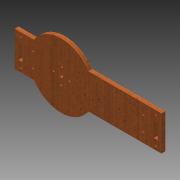
# Autodesk Inventor part: tiltStructureCrossBeamRB01
Saved by Autodesk Inventor 2013 (Build 170138000, 138)
## iProperties
Created: 2014-06-14
Part Number: tiltStructureCrossBeamRB01
Material: Wood (Cherry)
Document SubType Name: Modeling
Designer: Byron
Density: 0.5 g/cm^3
Mass: 49.6326 g
Surface Area: 357.646 cm^2
Volume: 99.2651 cm^3
Author: Byron
Autodesk Inventor part; units mm, degrees
ref_plane "YZ Plane" through (0, 0, 0) normal (1, 0, 0) x (0, 1, 0)
ref_plane "XZ Plane" through (0, 0, 0) normal (0, 1, 0) x (-1, 0, 0)
ref_plane "XY Plane" through (0, 0, 0) normal (0, 0, 1) x (1, 0, 0)
sketch "Sketch1" plane through (0, 0, 0) normal (0, 0, 1) x (1, 0, 0)
  line L0 (0, 78.0122) -> (0, 82.508) projected
  line L1 (-6.35, 82.508) -> (-6.35, 78.0122) projected
  line L2 (-6.35, 78.0122) -> (0, 78.0122) projected
  line L3 (222.25, 130.6664) -> (222.25, 135.1622) projected
  line L4 (215.9, 135.1622) -> (222.25, 135.1622) projected
  line L5 (215.9, 135.1622) -> (215.9, 130.6664) projected
  line L6 (222.25, 78.0122) -> (222.25, 135.1622)
  line L7 (-6.35, 135.1622) -> (-6.35, 78.0122)
  arc A0 (65.1726, 108.6235) -> (63.7223, 104.0872) centre (63.7223, 106.5872) ccw projected
  line L8 (222.25, 135.1622) -> (108.3945, 135.1622)
  line L9 (19.05, 135.1622) -> (-6.35, 135.1622)
  line L10 (-6.35, 78.0122) -> (19.05, 78.0122)
  line L11 (108.3945, 78.0122) -> (222.25, 78.0122)
  arc A1 (108.3945, 135.1622) -> (19.05, 135.1622) centre (63.7223, 106.5872) ccw
  arc A2 (19.05, 78.0122) -> (108.3945, 78.0122) centre (63.7223, 106.5872) ccw
  line L12 (215.9, 130.6664) -> (222.25, 130.6664) projected
  line L13 (0, 82.508) -> (-6.35, 82.508) projected
  point P0 (0, 0)
  dimension "d19" = 57.15
  dimension "d20" = 57.15
  dimension "d21" = 228.6
  dimension "d22" = 228.6
  dimension "d23" = 25.4
  dimension "d24" = 25.4
  dimension "d25" = 113.8555
  dimension "d26" = 113.8555
  constraints: 12 end point, 5 parallel, 4 point on circle, 2 centre point, 2 horizontal, 2 perpendicular, 1 coincident
  measures "d19" distance of L6.start L3.end
  measures "d20" distance of L7.start L1.end
  measures "d21" distance of L6.start L1.end
  measures "d22" distance of L3.end L7.start
  measures "d23" distance of L9.start L7.start
  measures "d24" distance of L1.end L10.end
  measures "d25" distance of L3.end L8.end
  measures "d26" distance of L11.start L6.start
extrude "Extrusion1" add sketch "Sketch1" along normal blind 6.35
sketch "Sketch2" plane through (0, 0, 0) normal (0, 0, -1) x (-1, 0, 0)
  line L0 (-53.2456, 114.8496) -> (-74.1989, 114.8496)
  line L1 (-13.716, 122.4622) -> (-13.716, 90.7122)
  line L2 (-63.7223, 114.8496) -> (-63.7223, 83.3208) construction
  line L3 (-13.716, 106.5872) -> (-74.4954, 106.5872) construction
  circle A0 centre (-63.7223, 106.5872) radius 3.175
  circle A1 centre (-63.1488, 93.4527) radius 1.8542
  circle A2 centre (-50.5878, 107.1607) radius 1.8542
  circle A3 centre (-64.2957, 119.7217) radius 1.8542
  circle A4 centre (-76.8567, 106.0138) radius 1.8542
  point P0 (0, 0)
extrude "Extrusion2" cut sketch "Sketch2" against normal through all
sketch "Sketch3" plane through (0, 0, 0) normal (0, 0, -1) x (-1, 0, 0)
  line L0 (6.35, 135.1622) -> (6.35, 78.0122) construction
  line L1 (-222.25, 135.1622) -> (-108.3945, 135.1622) construction
  line L2 (-222.25, 78.0122) -> (-222.25, 135.1622) construction
  line L3 (-108.3945, 78.0122) -> (-222.25, 78.0122) construction
  line L4 (-215.9, 135.1622) -> (-215.9, 130.6664) construction
  line L5 (-217.6131, 96.5879) -> (-200.4173, 96.5879) construction
  line L6 (-200.4173, 90.2379) -> (-217.6131, 90.2379) construction
  line L7 (-217.6131, 90.2379) -> (-217.6131, 96.5879) construction
  line L8 (-217.6131, 121.9879) -> (-200.4173, 121.9879) construction
  line L9 (-200.4173, 115.6379) -> (-217.6131, 115.6379) construction
  line L10 (-217.6131, 115.6379) -> (-217.6131, 121.9879) construction
  circle A0 centre (-219.075, 128.8122) radius 1.8542
  circle A1 centre (-198.5631, 118.6522) radius 1.8542
  line L11 (-222.25, 106.5872) -> (-215.9, 106.5872) construction
  circle A2 centre (-219.075, 84.3622) radius 1.8542
  circle A3 centre (-198.5631, 94.5222) radius 1.8542
  line L12 (-107.95, 135.1622) -> (-107.95, 78.0122) construction
  circle A4 centre (3.175, 128.8122) radius 1.8542
  circle A5 centre (-17.3369, 118.6522) radius 1.8542
  circle A6 centre (-17.3369, 94.5222) radius 1.8542
  circle A7 centre (3.175, 84.3622) radius 1.8542
  line L13 (-200.4173, 121.9879) -> (-200.4173, 115.6379) projected
  line L14 (-200.4173, 96.5879) -> (-200.4173, 90.2379) projected
  line L15 (6.35, 78.0122) -> (-19.05, 78.0122) projected
  line L16 (-19.05, 135.1622) -> (6.35, 135.1622) projected
  point P0 (0, 0)
  point P1 (-215.9, 135.1622)
  dimension "d7" = 3.7084
  dimension "d8" = 3.175
  dimension "d9" = 3.175
  dimension "d10" = 6.35
  dimension "d11" = 3.7084
  dimension "d12" = 19.05
  dimension "d13" = 28.575
  dimension "d14" = 28.575
  dimension "d15" = 114.3
  dimension "d16" = 114.3
  dimension "d27" = 16.51
  dimension "d28" = 16.51
  dimension "d29" = 23.6868
  dimension "d30" = 23.6868
  dimension "d31" = 16.51
  dimension "d32" = 16.51
  dimension "d33" = 23.6868
  dimension "d34" = 23.6868
  constraints: 8 centre point, 6 symmetric about line, 4 end point, 8 other
  measures "d7" diameter of A0
  measures "d8" distance from line of A0.centre L2
  measures "d10" distance from line of A0.centre L1
  measures "d11" diameter of A1
  measures "d12" distance from line of L10 A1.centre
  measures "d14" distance between parallel lines of L1 L11
  measures "d15" distance between parallel lines of L2 L12
  measures "d16" distance between parallel lines of L0 L12
  measures "d27" distance from line of L1 A1.centre
  measures "d29" distance from line of L2 A1.centre
  measures "d30" distance from line of L2 A3.centre
  measures "d31" distance from line of L16 A5.centre
  measures "d32" distance from line of L15 A6.centre
  measures "d33" distance from line of L0 A5.centre
  measures "d34" distance from line of L0 A6.centre
extrude "Extrusion3" cut sketch "Sketch3" against normal through all
sketch "Sketch4" plane through (0, 0, 6.35) normal (0, 0, 1) x (1, 0, 0)
  line L0 (222.25, 135.1622) -> (228.6, 135.1622)
  line L1 (228.6, 135.1622) -> (228.6, 78.0122)
  line L2 (228.6, 78.0122) -> (222.25, 78.0122)
  line L3 (222.25, 78.0122) -> (222.25, 135.1622)
  line L4 (-6.35, 78.0122) -> (-12.7, 78.0122)
  line L5 (-12.7, 78.0122) -> (-12.7, 135.1622)
  line L6 (-12.7, 135.1622) -> (-6.35, 135.1622)
  line L7 (-6.35, 135.1622) -> (-6.35, 78.0122)
  point P0 (0, 0)
  dimension "d35" = 6.35
  dimension "d36" = 57.15
  dimension "d37" = 6.35
  dimension "d38" = 57.15
  constraints: 16 end point, 4 parallel, 2 horizontal, 2 perpendicular
  measures "d35" distance of L1.end L2.end
  measures "d36" distance of L0.end L1.end
  measures "d37" distance of L5.end L6.end
  measures "d38" distance of L4.end L5.end
extrude "Extrusion4" add sketch "Sketch4" against normal blind 6.35
sketch "Sketch5" plane through (0, 0, 6.35) normal (0, 0, 1) x (1, 0, 0)
  line L0 (228.6, 135.1622) -> (228.6, 78.0122) projected
  line L1 (-12.7, 78.0122) -> (-12.7, 135.1622) projected
  line L2 (215.9, 125.1613) -> (215.9, 88.0132) projected
  line L3 (222.25, 88.0132) -> (215.9, 88.0132) projected
  line L4 (222.25, 88.0132) -> (222.25, 125.1613) projected
  line L5 (222.25, 125.1613) -> (215.9, 125.1613) projected
  line L6 (-6.35, 125.1613) -> (-6.35, 88.0132) projected
  line L7 (0, 88.0132) -> (-6.35, 88.0132) projected
  line L8 (0, 88.0132) -> (0, 125.1613) projected
  line L9 (0, 125.1613) -> (-6.35, 125.1613) projected
  line L10 (215.9, 119.2872) -> (222.25, 119.2872)
  line L11 (222.25, 119.2872) -> (222.25, 93.8872)
  line L12 (222.25, 93.8872) -> (215.9, 93.8872)
  line L13 (215.9, 93.8872) -> (215.9, 119.2872)
  line L14 (-12.7, 106.5872) -> (228.6, 106.5872) construction
  line L15 (107.95, 135.1622) -> (107.95, 78.0122) construction
  line L16 (-6.35, 125.1613) -> (0, 125.1613)
  line L17 (0, 119.2872) -> (-6.35, 119.2872)
  line L18 (-6.35, 119.2872) -> (-6.35, 93.8872)
  line L19 (-6.35, 93.8872) -> (0, 93.8872)
  line L20 (0, 93.8872) -> (0, 119.2872)
  point P0 (0, 0)
  dimension "d41" = 25.4
  dimension "d43" = 5.874
  dimension "d44" = 5.874
  dimension "d45" = 120.65
  dimension "d46" = 120.65
  constraints: 20 end point, 4 symmetric about line, 2 collinear, 2 parallel, 1 horizontal, 1 perpendicular
  measures "d41" distance of L10.end L11.end
  measures "d43" distance between parallel lines of L5 L10
  measures "d44" distance between parallel lines of L3 L12
  measures "d45" distance between parallel lines of L0 L15
  measures "d46" distance between parallel lines of L1 L15
extrude "Extrusion5" cut sketch "Sketch5" against normal through all contours L10 L4 L12 L2 | L17 L8 L19 L6
equation "\"d8\" = d9"
equation "\"d13\" = d14"
equation "\"d15\" = d16"
equation "\"d43\" = d44"
equation "\"d45\" = d46"
body "Solid1"
